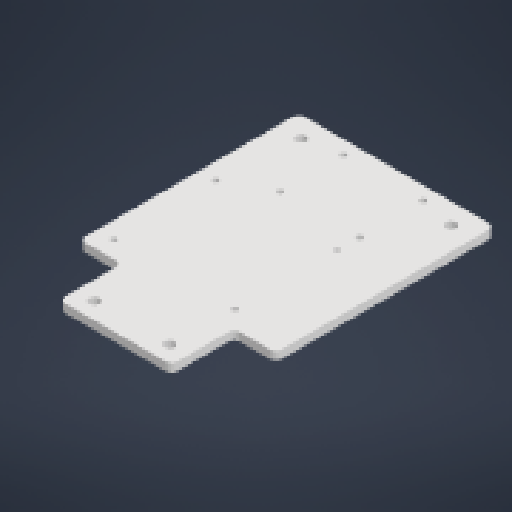
# Autodesk Inventor part: 1.5_base_2
Saved by Autodesk Inventor 2025 (Build 290162010, 162A)
## iProperties
Created: 2024-05-22
Part Number: 1.5_base_2
Material: Generic
Document SubType Name: Modeling
Designer: Garfieldcmix
Density: 1 g/cm^3
Appearance: Default
Author: Garfieldcmix
Autodesk Inventor part; units mm, degrees
ref_plane "YZ Plane" through (0, 0, 0) normal (1, 0, 0) x (0, 1, 0)
ref_plane "XZ Plane" through (0, 0, 0) normal (0, 1, 0) x (-1, 0, 0)
ref_plane "XY Plane" through (0, 0, 0) normal (0, 0, 1) x (1, 0, 0)
derived "Car_Plan.ipt"
sketch "Car_Sketch" plane through (0, 0, 0) normal (0, 1, 0) x (-1, 0, 0)
  line L0 (0, 0) -> (94, 0)
  line L1 (0, 0) -> (0, 105)
  line L2 (94, 0) -> (94, 105)
  line L3 (0, 105) -> (20, 105)
  line L4 (20, 105) -> (20, 190)
  line L5 (20, 190) -> (74, 190)
  line L6 (74, 190) -> (74, 105)
  line L7 (74, 105) -> (94, 105)
  line L8 (-5, 68) -> (-5, 0)
  line L9 (-5, 0) -> (-32, 0)
  line L10 (-32, 0) -> (-32, 68)
  line L11 (-32, 68) -> (-5, 68)
  line L12 (47, 190) -> (47, 0) construction
  line L13 (126, 68) -> (99, 68)
  line L14 (99, 68) -> (99, 0)
  line L15 (126, 0) -> (126, 68)
  line L16 (99, 0) -> (126, 0)
  line L17 (-5, 34) -> (99, 34) construction
  line L18 (0, 95) -> (94, 95) construction
  line L19 (-5, 190) -> (-32, 190)
  line L20 (-32, 122) -> (-5, 122)
  line L21 (-32, 190) -> (-32, 122)
  line L22 (-5, 122) -> (-5, 190)
  line L23 (-5, 156) -> (99, 156) construction
  line L24 (126, 122) -> (99, 122)
  line L25 (126, 190) -> (126, 122)
  line L26 (99, 190) -> (126, 190)
  line L27 (99, 122) -> (99, 190)
  line L28 (0, 156) -> (47, 34) construction
  line L29 (94, 156) -> (47, 34) construction
  line L30 (0, 156) -> (-174.2341, 34) construction
  line L31 (-5, 34) -> (-174.2341, 34) construction
  line L32 (8.9873, 132.6713) -> (47, 141.55) construction
  line L33 (85.0127, 132.6713) -> (47, 141.55) construction
sketch "Base" plane through (0, 0, 0) normal (0, 1, 0) x (-1, 0, 0)
  line L0 (0, 0) -> (0, 105) projected
  line L1 (0, 105) -> (20, 105) projected
  line L2 (20, 105) -> (20, 190) projected
  line L3 (74, 190) -> (74, 105) projected
  line L4 (74, 105) -> (94, 105) projected
  line L5 (94, 0) -> (94, 105) projected
  line L6 (0, 0) -> (94, 0) projected
  line L7 (74, 135) -> (20, 135)
  circle A0 centre (29, 127) radius 2.4
  circle A1 centre (65, 127) radius 2.4
  circle A2 centre (11.1, 10) radius 2.4
  circle A3 centre (82.9, 10) radius 2.4
  dimension "d76" = 30
  dimension "d77" = 4.8
  dimension "d78" = 4.8
  dimension "d79" = 9
  dimension "d80" = 22
  dimension "d81" = 22
  dimension "d82" = 9
  dimension "d83" = 4.8
  dimension "d84" = 4.8
  dimension "d85" = 10
  dimension "d86" = 11.1
  dimension "d87" = 10
  dimension "d88" = 11.1
  constraints: 4 centre point, 2 end point, 2 point on line, 1 perpendicular
  measures "d76" distance between parallel lines of L1 L7
  measures "d77" diameter of A0
  measures "d78" diameter of A1
  measures "d79" distance from line of L2 A0.centre
  measures "d80" distance from line of L1 A0.centre
  measures "d81" distance from line of A1.centre L4
  measures "d82" distance from line of L3 A1.centre
  measures "d83" diameter of A2
  measures "d84" diameter of A3
  measures "d85" distance from line of L6 A2.centre
  measures "d86" distance from line of L0 A2.centre
  measures "d87" distance from line of L6 A3.centre
  measures "d88" distance from line of L5 A3.centre
extrude "Extrusion1" add sketch "Base" along normal blind 4
fillet "Fillet2" radius 3 8 edges at (-20, 2, 105) (0, 2, 105) (0, 2, 0) (-94, 2, 0) (-94, 2, 105) (-74, 2, 105) (-74, 2, 135) (-20, 2, 135)
sketch "Sketch19" plane through (0, 4, 0) normal (0, 1, 0) x (1, 0, 0)
  line L0 (0, -102) -> (0, -3) projected
  line L1 (-17, -105) -> (-3, -105) projected
  line L2 (-94, -3) -> (-94, -102) projected
  line L3 (-91, -105) -> (-77, -105) projected
  line L4 (0, -70) -> (-4.5, -70)
  line L5 (-4.5, -70) -> (-89.5, -70)
  line L6 (-89.5, -70) -> (-89.5, -14)
  line L7 (-89.5, -14) -> (-4.5, -14)
  line L8 (-4.5, -14) -> (-4.5, -70)
  line L9 (-4.5, -70) -> (-8, -70)
  line L10 (-4.5, -66.5) -> (-4.5, -70)
  circle A0 centre (-28, -66.5) radius 1.25
  line L11 (-28, -66.5) -> (-24.5, -66.5)
  line L12 (-24.5, -66.5) -> (-24.5, -70)
  line L13 (-24.5, -70) -> (-28, -70)
  line L14 (-28, -70) -> (-28, -66.5)
  line L15 (-24.5, -70) -> (-89.5, -70)
  line L16 (-89.5, -70) -> (-89.5, -14)
  line L17 (-89.5, -14) -> (-24.5, -14)
  line L18 (-24.5, -14) -> (-24.5, -70)
  line L19 (-57, -70) -> (-57, -56.7745)
  line L20 (-24.5, -42) -> (-39.3063, -42)
  circle A1 centre (-86, -66.5) radius 1.25
  circle A2 centre (-28, -17.5) radius 1.25
  circle A3 centre (-86, -17.5) radius 1.25
  point P0 (0, 0)
  dimension "d196" = 4.5
  dimension "d197" = 85
  dimension "d198" = 56
  dimension "d199" = 35
  dimension "d202" = 2.5
  dimension "d203" = 3.5
  dimension "d204" = 23.5
  dimension "d205" = 3.5
  constraints: 34 end point, 6 horizontal, 6 parallel, 4 centre point, 3 perpendicular, 3 symmetric about line, 2 midpoint, 2 point on line, 1 vertical, 3 other
  measures "d196" distance of L4.start L4.end
  measures "d197" distance of L6.end L7.end
  measures "d198" distance of L5.end L6.end
  measures "d199" distance between parallel lines of L1 L4
  measures "d202" diameter of A0
  measures "d203" distance from line of L5 L11.start
  measures "d204" distance from line of L8 L11.start
  measures "d205" distance of L12.end L13.end
extrude "Extrusion12" cut sketch "Sketch19" against normal through all contours L14 L11 A0 | A0 L11 L14 | A1 | A2 | A3
sketch "Sketch20" plane through (0, 4, 0) normal (0, 1, 0) x (1, 0, 0)
  line L0 (0, -102) -> (0, -3) projected
  line L1 (0, -80) -> (-25.4, -80)
  line L2 (-3, 0) -> (-91, 0) projected
  line L3 (-25.4, -80) -> (-68.58, -80)
  line L4 (-68.58, -80) -> (-68.58, -115.56)
  line L5 (-68.58, -115.56) -> (-25.4, -115.56)
  line L6 (-25.4, -115.56) -> (-25.4, -80)
  line L7 (-25.4, -115.56) -> (-27.94, -115.56)
  line L8 (-27.94, -115.56) -> (-27.94, -113.02)
  line L9 (-27.94, -113.02) -> (-25.4, -113.02)
  line L10 (-25.4, -113.02) -> (-25.4, -115.56)
  circle A0 centre (-27.94, -113.02) radius 1.5
  line L11 (-46.99, -115.56) -> (-46.99, -107.0811)
  line L12 (-25.4, -97.78) -> (-34.7805, -97.78)
  circle A1 centre (-66.04, -113.02) radius 1.5
  circle A2 centre (-27.94, -82.54) radius 1.5
  circle A3 centre (-66.04, -82.54) radius 1.5
  line L13 (-68.58, -80) -> (-59.88, -80)
  line L14 (-59.88, -80) -> (-59.88, -84.4)
  line L15 (-59.88, -84.4) -> (-68.58, -84.4)
  line L16 (-68.58, -84.4) -> (-68.58, -80)
  line L17 (-59.88, -84.4) -> (-32.88, -84.4)
  line L18 (-32.88, -84.4) -> (-32.88, -85.9)
  line L19 (-32.88, -85.9) -> (-59.88, -85.9)
  line L20 (-59.88, -85.9) -> (-59.88, -84.4)
  point P0 (0, 0)
  dimension "d208" = 25.4
  dimension "d209" = 80
  dimension "d210" = 43.18
  dimension "d211" = 35.56
  dimension "d212" = 2.54
  dimension "d213" = 2.54
  dimension "d214" = 3
  dimension "d231" = 8.7
  dimension "d232" = 4.4
  dimension "d233" = 27
  dimension "d234" = 1.5
  constraints: 38 end point, 8 parallel, 5 horizontal, 5 perpendicular, 4 centre point, 3 symmetric about line, 2 midpoint, 1 coincident, 1 point on line, 1 vertical, 3 other
  measures "d208" distance of L1.start L1.end
  measures "d209" distance between parallel lines of L2 L1
  measures "d210" distance of L5.end L4.end
  measures "d211" distance of L4.end L3.end
  measures "d212" distance of L8.end L9.end
  measures "d213" distance of L7.end L8.end
  measures "d214" diameter of A0
  measures "d231" distance of L14.end L15.end
  measures "d232" distance of L13.end L14.end
  measures "d233" distance of L18.end L19.end
  measures "d234" distance of L17.end L18.end
extrude "Extrusion13" cut sketch "Sketch20" against normal through all contours L17 L18 L19 L20 | A0 L8 L9 | L9 L8 A0 | A1 | A2 | A3
sketch "Sketch21" plane through (0, 4, 0) normal (0, 1, 0) x (1, 0, 0)
  line L0 (-4.5, -70) -> (-91.5586, -70)
  line L1 (-89.5, -14) -> (-4.5, -14)
  line L2 (-4.5, -14) -> (-4.5, -70)
  line L3 (-24.5, -70) -> (-89.5, -70)
  line L4 (-89.5, -70) -> (-89.5, -14)
  line L5 (-89.5, -14) -> (-24.5, -14)
  line L6 (-24.5, -14) -> (-24.5, -70)
  line L7 (0, -102) -> (0, -3) projected
  line L8 (-17, -105) -> (-3, -105) projected
  line L9 (-3, 0) -> (-91, 0) projected
  line L10 (-24.5, -70) -> (-28, -70)
  line L11 (-28, -70) -> (-28, -66.5)
  line L12 (-28, -66.5) -> (-24.5, -66.5)
  line L13 (-24.5, -66.5) -> (-24.5, -70)
  circle A0 centre (-28, -66.5) radius 2.5
  line L14 (-57, -70) -> (-57, -55.9605)
  line L15 (-24.5, -42) -> (-45.4996, -42)
  circle A1 centre (-86, -66.5) radius 2.5
  circle A2 centre (-28, -17.5) radius 2.5
  circle A3 centre (-86, -17.5) radius 2.5
  circle A4 centre (-28, -66.5) radius 1.35
  circle A5 centre (-86, -66.5) radius 1.35
  circle A6 centre (-28, -17.5) radius 1.35
  circle A7 centre (-86, -17.5) radius 1.35
  point P0 (0, 0)
  dimension "d217" = 85
  dimension "d219" = 4.5
  dimension "d220" = 35
  dimension "d221" = 20
  dimension "d223" = 56
  dimension "d224" = 65
  dimension "d225" = 3.5
  dimension "d226" = 3.5
  dimension "d227" = 5
  dimension "d228" = 2.7
  constraints: 26 end point, 8 centre point, 6 symmetric about line, 5 parallel, 4 horizontal, 2 coincident, 2 midpoint, 2 perpendicular, 1 point on line, 1 vertical, 6 other
  measures "d217" distance of L5.start L2.start
  measures "d219" distance between parallel lines of L7 L2
  measures "d220" distance between parallel lines of L8 L0
  measures "d221" distance between parallel lines of L2 L6
  measures "d223" distance between parallel lines of L3 L5
  measures "d224" distance between parallel lines of L4 L6
  measures "d225" distance of L11.end L12.end
  measures "d226" distance of L10.end L11.end
  measures "d227" diameter of A0
  measures "d228" diameter of A4
extrude "Extrusion14" add sketch "Sketch21" along normal blind 2.5 contours A0 L12 A4 L11 | L11 A4 L12 A0 | A1 | A2 | A3
body "Solid1"
